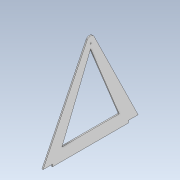
# Autodesk Inventor part: Stand
Saved by Autodesk Inventor 2021 (Build 250183000, 183)
## iProperties
Created: 2021-08-28
Part Number: Stand
Material: Generic
Document SubType Name: Modeling
Designer: digge
Density: 1 g/cm^3
Appearance: Default
Author: digge
Autodesk Inventor part; units mm, degrees
ref_plane "YZ Plane" through (0, 0, 0) normal (1, 0, 0) x (0, 1, 0)
ref_plane "XZ Plane" through (0, 0, 0) normal (0, 1, 0) x (-1, 0, 0)
ref_plane "XY Plane" through (0, 0, 0) normal (0, 0, 1) x (1, 0, 0)
sketch "Sketch1" plane through (0, 0, 0) normal (1, 0, 0) x (0, 1, 0)
  line L0 (12, 259.0874) -> (12, 234.0874)
  line L1 (12, 234.0874) -> (6, 234.0874)
  line L2 (6, 234.0874) -> (6, 34.0874)
  line L3 (6, 34.0874) -> (12, 34.0874)
  line L4 (12, 34.0874) -> (12, 9.0874)
  line L5 (12, 9.0874) -> (267, 134.0874)
  line L6 (267, 134.0874) -> (12, 259.0874)
  circle A0 centre (237, 134.0874) radius 1.5
  line L7 (267, 134.0874) -> (6, 134.0874) construction
  point P0 (0, 0)
  dimension "d0" = 3
  dimension "d1" = 6
  dimension "d2" = 200
  dimension "d4" = 30
  dimension "d5" = 250
  dimension "d8" = 255
  dimension "d9" = 225
  constraints: 16 end point, 3 perpendicular, 3 point on line, 1 centre point, 1 midpoint, 1 vertical, 2 other
  measures "d0" diameter of A0
  measures "d1" distance of L0.end L1.end
  measures "d2" distance of L1.end L2.end
  measures "d4" distance of L5.end A0.centre
  measures "d5" distance of L4.end L0.start
  measures "d8" distance from line of L0 L5.end
  measures "d9" distance from line of L0 A0.centre
extrude "Extrusion1" add sketch "Sketch1" along normal blind 3
fillet "Fillet1" radius 10 1 edges at (1.5, 267, 134.0874)
sketch "Sketch2" plane through (0, 0, 0) normal (-1, 0, 0) x (0, 0, 1)
  line L0 (58.6161, 38.8141) -> (209.5588, 38.8141)
  line L1 (209.5588, 38.8141) -> (134.0874, 224.8352)
  line L2 (134.0874, 224.8352) -> (58.6161, 38.8141)
  line L3 (234.0874, 6) -> (34.0874, 6) projected
  circle A0 centre (134.0874, 237) radius 1.5 projected
  line L4 (134.0874, 237) -> (134.0874, 6) construction
  line L5 (234.0874, 6) -> (34.0874, 6) projected
  point P0 (0, 0)
  constraints: 8 end point, 1 horizontal, 1 midpoint, 1 point on line, 1 other
extrude "Extrusion2" cut sketch "Sketch2" against normal blind 3 contours L2 L1 L0
equation "\"d0\" = ScrewDiameter"
equation "\"d1\" = 2 * Width"
equation "\"d2\" = SlotLength"
equation "\"d4\" = HingeDistance"
equation "\"d5\" = StandWidth"
equation "\"d8\" = WheelClearance + 0.5 * WheelDiameter + HingeDistance"
equation "\"d10\" = Width"
equation "\"d13\" = Width"
equation "\"ScrewDiameter\" = 3"
equation "\"Width\" = 3"
equation "\"SlotLength\" = 200"
equation "\"HingeDistance\" = 30"
equation "\"StandWidth\" = 250"
equation "\"WheelClearance\" = 100"
equation "\"WheelDiameter\" = 250"
body "Solid1"
